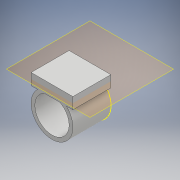
# Autodesk Inventor part: bague
Saved by Autodesk Inventor 2018 (Build 220112000, 112)
## iProperties
Created: 2018-04-09
Part Number: bague
Material: Générique
Document SubType Name: Modeling
Designer: Dimitri
Density: 1 g/cm^3
Appearance: Par défaut
Author: Dimitri
Autodesk Inventor part; units mm, degrees
ref_plane "YZ Plane" through (0, 0, 0) normal (1, 0, 0) x (0, 1, 0)
ref_plane "XZ Plane" through (0, 0, 0) normal (0, 1, 0) x (-1, 0, 0)
ref_plane "XY Plane" through (0, 0, 0) normal (0, 0, 1) x (1, 0, 0)
sketch "Esquisse1" plane through (0, 0, 0) normal (0, 1, 0) x (-1, 0, 0)
  circle A0 centre (0, 0) radius 4.5
  circle A1 centre (0, 0) radius 5.5
  dimension "d0" = 9
  dimension "d1" = 11
  constraints: 2 centre point, 2 coincident
  measures "d0" diameter of A0
  measures "d1" diameter of A1
extrude "Extrusion1" add sketch "Esquisse1" along normal blind 10
sketch "Esquisse2" plane through (0, 10, 0) normal (0, 1, 0) x (1, 0, 0)
  circle A0 centre (0, 0) radius 5.5 projected
  point P0 (0, -5.5)
  constraints: 1 vertical alignment, 1 other
ref_plane "Plan de construction1" through (0, 10, 5.5) normal (0, 0, 1) x (1, 0, 0)
sketch "Esquisse3" plane through (0, 10, 5.5) normal (0, 0, 1) x (1, 0, 0)
  line L0 (-5.5, -10) -> (-5.5, 0) projected
  line L1 (-5.5, -10) -> (5.5, -10) projected
  line L2 (-5.5, 0) -> (5.5, 0)
  line L3 (5.5, 0) -> (5.5, -10)
  line L4 (5.5, -10) -> (-5.5, -10)
  line L5 (-5.5, -10) -> (-5.5, 0)
  point P0 (0, -10)
  constraints: 8 end point, 2 parallel, 1 horizontal, 1 perpendicular, 1 point on line
extrude "Extrusion2" add sketch "Esquisse3" along normal mid plane 3
